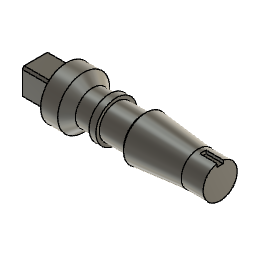
Shaft01 (Autodesk Fusion 360 design; units mm, degrees)
Autodesk Fusion 360 part; units mm, degrees
sketch "Sketch1" plane through (0, 0, 0) normal (0, 1, 0) x (1, 0, 0) in component "Shaft"
  line L0 (0, 0) -> (25, 0)
  line L1 (25, 38) -> (0, 38)
  line L2 (0, 38) -> (0, 0)
  line L3 (25, 38) -> (38, 25)
  line L4 (38, 25) -> (63, 25)
  line L5 (63, 25) -> (63, 30)
  line L6 (63, 30) -> (73, 30)
  line L7 (73, 30) -> (73, 25)
  line L8 (73, 25) -> (113, 25)
  line L9 (113, 25) -> (113, 32.5)
  line L10 (113, 32.5) -> (116, 32.5)
  line L11 (0, 0) -> (193, 0)
  line L12 (116, 32.5) -> (193, 25)
  line L13 (193, 25) -> (225, 25)
  line L14 (225, 25) -> (225, 0)
  line L15 (225, 0) -> (193, 0)
  dimension "d2" = 25
  dimension "d3" = 38
  dimension "d8" = 25
  dimension "d9" = 5
  dimension "d10" = 10
  dimension "d11" = 5
  dimension "d12" = 13
  dimension "d13" = 40
  dimension "d15" = 3
  dimension "d17" = 25
  dimension "d18" = 32
  constraint horizontal L0
  constraint horizontal L1
  constraint vertical L2
  constraint coincident L0.start L2.end
  constraint perpendicular L4 L5
  constraint perpendicular L5 L6
  constraint perpendicular L6 L7
  constraint perpendicular L7 L8
  constraint vertical L9
  constraint perpendicular L9 L10
  constraint perpendicular L2 L11
  measures "d2" distance of L1.start L1.end
  measures "d3" distance of L0.end L1.start
  measures "d8" distance of L3.end L4.end
  measures "d9" distance of L4.end L5.end
  measures "d10" distance of L5.end L6.end
  measures "d11" distance of L6.end L7.end
  measures "d12" horizontal distance of L1.start L3.end
  measures "d13" distance of L7.end L8.end
  measures "d15" distance of L9.end L10.end
  measures "d17" distance of L11.end L12.end
  measures "d18" distance of L12.end L13.end
revolve "Revolve1" add sketch "Sketch1" angle 360 about axis through (0, 0, 0) along (1, 0, 0) in component "Shaft"
sketch "Sketch2" plane through (0, 0, 0) normal (-1, 0, 0) x (0, -1, 0) in component "Shaft"
  circle A0 centre (0, 0) radius 38
  line L0 (20, -20) -> (-20, -20)
  line L1 (-20, -20) -> (-20, 20)
  line L2 (-20, 20) -> (20, 20)
  line L3 (20, 20) -> (20, -20)
  line L4 (20, -20) -> (-20, 20) construction
  line L5 (-20, -20) -> (20, 20) construction
  dimension "d20" = 40
  dimension "d21" = 40
  constraint horizontal L0
  constraint perpendicular L0 L1
  constraint parallel L0 L2
  constraint parallel L1 L3
  constraint coincident L4 A0.centre
  constraint coincident L5 A0.centre
  constraint coincident A0.centre origin
  measures "d20" distance of L1.end L2.end
  measures "d21" distance of L0.end L1.end
extrude "Extrude1" add sketch "Sketch2" along normal blind 45 contours L0 L1 L2 L3 in component "Shaft"
sketch "Sketch3" plane through (225, 0, 0) normal (1, 0, 0) x (0, 1, 0) in component "Shaft"
  circle A0 centre (0, 0) radius 25
  circle A1 centre (0, 0) radius 25
  line L0 (4.5, 20) -> (-4.5, 20)
  arc A2 (4.5, 24.5917) -> (-4.5, 24.5917) centre (0, 0) ccw
  line L1 (4.5, 20) -> (4.5, 24.5917)
  line L2 (-4.5, 20) -> (-4.5, 24.5917)
  constraint coincident A0 A2.end
extrude "Extrude2" cut sketch "Sketch3" against normal blind 25 contours A0 A1 L0 A2 L1 L2 in component "Shaft"
chamfer "Chamfer1" distance 3 angle 45 5 edges at (-22.5, -20, 20) (-22.5, 20, 20) (-22.5, -20, -20) (-22.5, 20, -20) (113, -11.7525, 30.3006) in component "Shaft"
component "Shaft" placed x (1, 0, 0) y (0, 1, 0) z (0, 0, 1) at (0, 0, 0)
